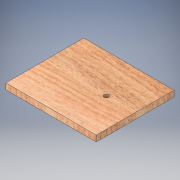
# Autodesk Inventor part: Stage2Wall
Saved by Autodesk Inventor 2017 (Build 210142000, 142)
## iProperties
Created: 2017-02-01
Part Number: Stage2Wall
Material: Wood (Birch)
Document SubType Name: Modeling
Designer: Naga
Density: 0.55 g/cm^3
Appearance: Birch - Natural Polished
Author: Naga
Autodesk Inventor part; units mm, degrees
ref_plane "YZ Plane" through (0, 0, 0) normal (1, 0, 0) x (0, 1, 0)
ref_plane "XZ Plane" through (0, 0, 0) normal (0, 1, 0) x (-1, 0, 0)
ref_plane "XY Plane" through (0, 0, 0) normal (0, 0, 1) x (1, 0, 0)
sketch "Sketch1" plane through (0, 0, 0) normal (0, 1, 0) x (-1, 0, 0)
  line L0 (0, 0) -> (-177.0062, 0)
  line L1 (-177.0062, 0) -> (-177.0062, -152.4)
  line L2 (-177.0062, -152.4) -> (0, -152.4)
  line L3 (0, -152.4) -> (0, 0)
  dimension "d0" = 177.0062
  dimension "d1" = 152.4
  constraints: 8 end point, 2 parallel, 1 horizontal, 1 perpendicular
  measures "d0" distance of L2.end L1.end
  measures "d1" distance of L0.end L1.end
extrude "Extrusion1" add sketch "Sketch1" along normal blind 11.9062
sketch "Sketch2" plane through (0, 11.9062, 0) normal (0, 1, 0) x (1, 0, 0)
  line L0 (0, 0) -> (177.0062, 0) projected
  line L1 (177.0062, 0) -> (177.0062, 152.4) projected
  line L2 (177.0062, 152.4) -> (0, 152.4) projected
  line L3 (0, 152.4) -> (0, 0) projected
  line L4 (0, 0) -> (177.0062, 0) projected
  line L5 (177.0062, 76.2) -> (120.65, 76.2)
  circle A0 centre (120.65, 76.2) radius 4.7625
  dimension "d4" = 56.3563
  dimension "d5" = 9.525
  constraints: 2 end point, 1 centre point, 1 coincident, 1 horizontal, 1 midpoint
  measures "d4" distance of L5.start L5.end
  measures "d5" diameter of A0
extrude "Extrusion2" cut sketch "Sketch2" against normal up to surface (11.9062 mm away) contours A0
body "Solid1"
